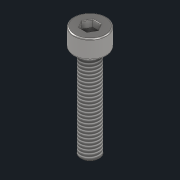
# Autodesk Inventor part: M4-20
Saved by Autodesk Inventor 2021 (Build 250183000, 183)
## iProperties
Created: 2021-06-08
Part Number: M4-20
Material: Steel, Carbon
Document SubType Name: Modeling
Designer: arbra
Density: 7.85 g/cm^3
Appearance: Semi-Polished
Author: arbra
Autodesk Inventor part; units mm, degrees
ref_plane "YZ Plane" through (0, 0, 0) normal (1, 0, 0) x (0, 1, 0)
ref_plane "XZ Plane" through (0, 0, 0) normal (0, 1, 0) x (-1, 0, 0)
ref_plane "XY Plane" through (0, 0, 0) normal (0, 0, 1) x (1, 0, 0)
sketch "Sketch1" plane through (0, 0, 0) normal (0, 1, 0) x (-1, 0, 0)
  circle A0 centre (0, 0) radius 3.5
  dimension "d0" = 7
  constraints: 1 centre point, 1 coincident
  measures "d0" diameter of A0
extrude "Extrusion1" add sketch "Sketch1" against normal blind 4
sketch "Sketch2" plane through (0, -4, 0) normal (0, -1, 0) x (1, 0, 0)
  circle A0 centre (0, 0) radius 2
  dimension "d3" = 4
  constraints: 1 centre point, 1 coincident
  measures "d3" diameter of A0
extrude "Extrusion2" add sketch "Sketch2" along normal blind 20
sketch "Sketch3" plane through (0, 0, 0) normal (0, 1, 0) x (1, 0, 0)
  circle A0 centre (0, 0) radius 2 construction
  line L0 (1.7321, 0) -> (0.866, -1.5)
  line L1 (0.866, -1.5) -> (-0.866, -1.5)
  line L2 (-0.866, -1.5) -> (-1.7321, 0)
  line L3 (-1.7321, 0) -> (-0.866, 1.5)
  line L4 (-0.866, 1.5) -> (0.866, 1.5)
  line L5 (0.866, 1.5) -> (1.7321, 0)
  dimension "d8" = 3
  constraints: 12 end point, 1 coincident, 1 horizontal, 13 other
  measures "d8" distance between parallel lines of L1 L4
extrude "Extrusion3" cut sketch "Sketch3" against normal blind 1.5
chamfer "Chamfer1" distance 0.25 angle 45 1 edges at (-2, -24, 0)
fillet "Fillet1" radius 0.25 2 edges at (3.5, 0, 0) (3.5, -4, 0)
chamfer "Chamfer2" distance 0.1 angle 45 6 edges at (0, 0, -1.5) (1.299, 0, -0.75) (1.299, 0, 0.75) (0, 0, 1.5) (-1.299, 0, 0.75) (-1.299, 0, -0.75)
thread "Thread2" size "M4x0.7" class "6g" standard "ANSI Metric M Profile" full length
body "Solid1"
